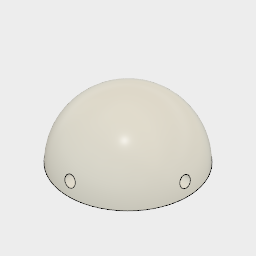
Battery Tube Dome (Autodesk Fusion 360 design; units mm, degrees)
Autodesk Fusion 360 part; units mm, degrees
sketch "Sketch1" plane through (0, 0, 0) normal (0, 1, 0) x (1, 0, 0)
  circle A0 centre (0, 0) radius 44.45
  dimension "d1" = 88.9
  measures "d1" diameter of A0
sketch "Sketch2" plane through (0, 0, 0) normal (0, 0, 1) x (1, 0, 0)
  line L0 (0, 0) -> (0, 44.45)
  arc A0 (44.45, 0) -> (0, 44.45) centre (0, 0) ccw
  line L1 (44.45, 0) -> (0, 0)
  line L2 (0, 0) -> (0, 38.1)
  arc A1 (38.1, 0) -> (0, 38.1) centre (0, 0) ccw
  line L3 (38.1, 0) -> (44.45, 0)
  dimension "d2" = 44.45
  dimension "d3" = 38.1
  measures "d2" distance of L0.start L0.end
  measures "d3" distance of L0.start L2.end
sweep "Sweep1" add profiles "Sketch2" path "Sketch1" along A0 section 1 contours L0 A0 L1 A1 L3
sketch "Sketch3" plane through (0, 0, 0) normal (0, 1, 0) x (1, 0, 0)
  line L0 (0, 0) -> (6.35, 0)
  line L1 (6.35, 0) -> (6.35, -6.35)
  line L2 (6.35, -6.35) -> (0, -6.35)
  line L3 (0, -6.35) -> (0, 0)
ref_plane "WorkPlane1" through (46.99, -3.175, 3.175) normal (1, 0, 0) x (0, 0, 1)
sketch "Sketch4" plane through (46.99, -3.175, 3.175) normal (1, 0, 0) x (0, 0, -1)
  line L0 (47.625, 3.175) -> (-41.275, 3.175)
  line L1 (0, 0) -> (0, 12.7)
  line L2 (0, 12.7) -> (2.54, 12.7)
  circle A0 centre (2.54, 12.7) radius 3.81
extrude "Extrude2" cut sketch "Sketch4" against normal blind 137.16
ref_plane "WorkPlane2" through (3.175, -3.175, 46.99) normal (0, 0, 1) x (-1, 0, 0)
sketch "Sketch5" plane through (3.175, -3.175, 46.99) normal (0, 0, 1) x (1, 0, 0)
  line L0 (3.175, 3.175) -> (-3.175, 3.175)
  line L1 (0, 0) -> (0, 12.7)
  line L2 (0, 12.7) -> (-3.175, 12.7)
  circle A0 centre (-3.175, 12.7) radius 3.81
  dimension "d14" = 7.62
  measures "d14" diameter of A0
extrude "Extrude3" cut sketch "Sketch5" against normal blind 129.54
